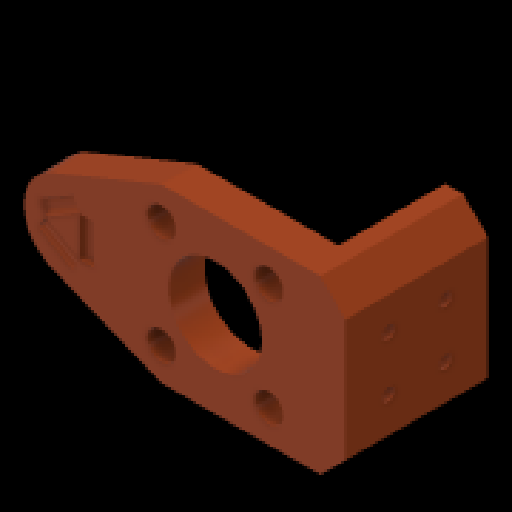
# Autodesk Inventor part: Rear Z Axis Carriage
Saved by Autodesk Inventor 2023.2 (Build 272271000, 271)
## iProperties
Created: 2023-02-17
Part Number: Rear Z Axis Carriage
Material: ABS Plastic
Document SubType Name: Modeling
Designer: remop
Density: 1.06 g/cm^3
Appearance: Smooth - Light Orange
Author: remop
Autodesk Inventor part; units mm, degrees
ref_plane "YZ Plane" through (0, 0, 0) normal (1, 0, 0) x (0, 1, 0)
ref_plane "XZ Plane" through (0, 0, 0) normal (0, 1, 0) x (-1, 0, 0)
ref_plane "XY Plane" through (0, 0, 0) normal (0, 0, 1) x (1, 0, 0)
sketch "Sketch1" plane through (0, 0, 0) normal (0, 0, 1) x (1, 0, 0)
  arc A0 (18.1843, -16.5324) -> (18.7618, -13.101) centre (16.0629, -14.4111) ccw projected
  arc A1 (18.7618, 13.101) -> (18.7618, -13.101) centre (45.75, 0) ccw projected
  arc A2 (18.7618, 13.101) -> (18.1843, 16.5324) centre (16.0629, 14.4111) ccw projected
  line L0 (11.5324, 23.1843) -> (18.1843, 16.5324) projected
  arc A3 (11.5324, 23.1843) -> (8.101, 23.7618) centre (9.4111, 21.0629) ccw projected
  arc A4 (-18.101, 23.7618) -> (8.101, 23.7618) centre (-5, 50.75) ccw projected
  arc A5 (-18.101, 23.7618) -> (-21.5324, 23.1843) centre (-19.4111, 21.0629) ccw projected
  line L1 (-28.1843, 16.5324) -> (-21.5324, 23.1843) projected
  arc A6 (-28.1843, 16.5324) -> (-28.7618, 13.101) centre (-26.0629, 14.4111) ccw projected
  arc A7 (-28.7618, -13.101) -> (-28.7618, 13.101) centre (-55.75, 0) ccw projected
  arc A8 (-28.7618, -13.101) -> (-28.1843, -16.5324) centre (-26.0629, -14.4111) ccw projected
  line L2 (-21.5324, -23.1843) -> (-28.1843, -16.5324) projected
  arc A9 (-21.5324, -23.1843) -> (-18.101, -23.7618) centre (-19.4111, -21.0629) ccw projected
  arc A10 (8.101, -23.7618) -> (-18.101, -23.7618) centre (-5, -50.75) ccw projected
  arc A11 (8.101, -23.7618) -> (11.5324, -23.1843) centre (9.4111, -21.0629) ccw projected
  line L3 (18.1843, -16.5324) -> (11.5324, -23.1843) projected
  circle A12 centre (10, -15) radius 4 projected
  circle A13 centre (-20, -15) radius 4 projected
  circle A14 centre (-20, 15) radius 4 projected
  circle A15 centre (10, 15) radius 4 projected
  circle A16 centre (-5, 0) radius 13 projected
  line L4 (39.4645, -4.5) -> (34.9645, -4.5) projected
  line L5 (34.9645, -4.5) -> (34.9645, 4.5) projected
  line L6 (34.9645, 4.5) -> (39.4645, 4.5) projected
  line L7 (39.4645, 4.5) -> (39.4645, 10) projected
  line L8 (39.4645, 10) -> (31.4645, 10) projected
  line L9 (31.4645, 10) -> (31.4645, -10) projected
  line L10 (31.4645, -10) -> (39.4645, -10) projected
  line L11 (39.4645, -10) -> (39.4645, -4.5) projected
  line L12 (31.4645, -10) -> (31.4645, -17.0711)
  line L13 (31.4645, -17.0711) -> (24.4726, -24.0629)
  line L14 (31.4645, 10) -> (31.4645, 17.0711)
  line L15 (-19.4111, -24.0629) -> (24.4726, -24.0629)
  line L16 (-19.4111, 24.0629) -> (24.4726, 24.0629)
  line L17 (31.4645, 17.0711) -> (24.4726, 24.0629)
  circle A17 centre (-46, 0) radius 12.5
  line L18 (-20.5407, -23.8421) -> (-50.7071, -11.5799)
  line L19 (-50.7071, 11.5799) -> (-20.5407, 23.8421)
  point P0 (0, 0)
  dimension "d0" = 45
  dimension "d1" = 5
  dimension "d4" = 46
  dimension "d5" = 25
  constraints: 16 end point, 8 tangent, 6 point on circle, 3 equal length, 2 vertical, 1 centre point, 1 horizontal alignment, 1 point on line
  measures "d0" angle of L12 L13
  measures "d1" distance from line of L9.end L13
  measures "d4" distance of A17.centre point (0, 0)
  measures "d5" diameter of A17
extrude "Extrusion1" add sketch "Sketch1" along normal blind 10 contours L3 A11 A10 A9 L2 A8 A7 A6 L1 A5 A4 A3 L0 A2 A1 A0 | A0 A1 A2 L0 A3 L16 L17 L14 L9 L12 L13 L15 A11 L3 | L15 A9 A10 A11 | L18 A17 L19 A5 L1 A6 A7 A8 L2 A9 | A3 A4 A5 L16 | A17
sketch "Sketch2" plane through (0, 0, 0) normal (0, 0, -1) x (-1, 0, 0)
  line L0 (-24.4726, -24.0629) -> (-31.4645, -17.0711) projected
  line L1 (19.4111, -24.0629) -> (-24.4726, -24.0629) projected
  arc A0 (19.4111, -24.0629) -> (20.5407, -23.8421) centre (19.4111, -21.0629) ccw projected
  line L2 (50.7071, -11.5799) -> (20.5407, -23.8421) projected
  arc A1 (50.7071, -11.5799) -> (50.7071, 11.5799) centre (46, 0) ccw projected
  line L3 (20.5407, 23.8421) -> (50.7071, 11.5799) projected
  arc A2 (20.5407, 23.8421) -> (19.4111, 24.0629) centre (19.4111, 21.0629) ccw projected
  line L4 (-24.4726, 24.0629) -> (19.4111, 24.0629) projected
  line L5 (-31.4645, 17.0711) -> (-24.4726, 24.0629) projected
  line L6 (-31.4645, -17.0711) -> (-31.4645, 17.0711) projected
  circle A3 centre (-10, -15) radius 4 projected
  circle A4 centre (20, -15) radius 4 projected
  circle A5 centre (20, 15) radius 4 projected
  circle A6 centre (-10, 15) radius 4 projected
  circle A7 centre (5, 0) radius 13 projected
  line L7 (-31.4645, 17.0711) -> (-23.4645, 17.0711)
  line L8 (-23.4645, 17.0711) -> (-23.4645, -17.0711)
  line L9 (-24.4726, -24.0629) -> (-31.4645, -17.0711) projected
  line L10 (-23.4645, -17.0711) -> (-31.4645, -17.0711)
  line L11 (-23.4645, 17.0711) -> (-19.4726, 21.0629)
  line L12 (-19.4726, 21.0629) -> (-19.4726, 24.0629)
  line L13 (-23.4645, -17.0711) -> (-19.4726, -21.0629)
  line L14 (-19.4726, -21.0629) -> (-19.4726, -24.0629)
  line L15 (19.4111, -24.0629) -> (-24.4726, -24.0629) projected
  point P0 (0, 0)
  dimension "d6" = 8
  dimension "d9" = 3
  constraints: 14 end point, 3 perpendicular, 3 point on line, 2 horizontal, 1 parallel, 1 vertical
  measures "d6" distance of L5.start L7.end
  measures "d9" distance of L11.end L12.end
extrude "Extrusion2" add sketch "Sketch2" along normal blind 29.9 contours L0 L10 L13 L14 L1 | L6 L7 L8 L10 | L5 L4 L12 L11 L7
sketch "Sketch3" plane through (23.4645, -17.0711, 0) normal (-1, 0, 0) x (0, 0, 1)
  line L0 (0, 34.1421) -> (0, 0) projected
  line L1 (0, 34.1421) -> (-29.9, 34.1421) projected
  line L2 (-29.9, 0) -> (-29.9, 34.1421) projected
  line L3 (0, 0) -> (-29.9, 0) projected
  point P0 (0, 17.0711)
  point P1 (-1.95, 25.0158)
  point P2 (-17.95, 25.0158)
  point P3 (-17.95, 10.0158)
  point P4 (-1.95, 10.0158)
  dimension "d10" = 15
  dimension "d11" = 16
  dimension "d12" = 11.95
  constraints: 2 horizontal alignment, 2 vertical alignment
  measures "d10" distance of point (-1.95, 10.016) point (-1.95, 25.016)
  measures "d11" distance of point (-17.95, 25.016) point (-1.95, 25.016)
  measures "d12" distance from line of L2 point (-17.95, 25.016)
hole "Hole1" at (23.4645, 7.9447, -1.95) at (23.4645, 7.9447, -17.95) at (23.4645, -7.0553, -17.95) at (23.4645, -7.0553, -1.95) direction (1, 0, 0) diameter 3.6 end through all counterbore diameter 6.5 counterbore depth 3.4 clearance for "Socket Head Cap Screw DIN EN ISO 4762" size "M3" standard "DIN"
sketch "Sketch4" plane through (0, 0, 0) normal (0, 0, -1) x (-1, 0, 0)
  circle A0 centre (5, 0) radius 13 projected
  circle A1 centre (-10, 15) radius 4 projected
  circle A2 centre (20, 15) radius 4 projected
  circle A3 centre (20, -15) radius 4 projected
  circle A4 centre (-10, -15) radius 4 projected
  line L0 (-19.4726, 24.0629) -> (-19.4726, 21.0629) projected
  line L1 (-19.4726, 21.0629) -> (-23.4645, 17.0711) projected
  line L2 (-23.4645, 17.0711) -> (-23.4645, 10.5447) projected
  line L3 (-23.4645, 10.5447) -> (-23.4645, 5.3447) projected
  line L4 (-23.4645, 5.3447) -> (-23.4645, -4.4553) projected
  line L5 (-23.4645, -4.4553) -> (-23.4645, -9.6553) projected
  line L6 (-23.4645, -9.6553) -> (-23.4645, -17.0711) projected
  line L7 (-23.4645, -17.0711) -> (-19.4726, -21.0629) projected
  line L8 (-19.4726, -21.0629) -> (-19.4726, -24.0629) projected
  line L9 (19.4111, -24.0629) -> (-19.4726, -24.0629) projected
  arc A5 (19.4111, -24.0629) -> (20.5407, -23.8421) centre (19.4111, -21.0629) ccw projected
  line L10 (50.7071, -11.5799) -> (20.5407, -23.8421) projected
  arc A6 (50.7071, -11.5799) -> (50.7071, 11.5799) centre (46, 0) ccw projected
  line L11 (20.5407, 23.8421) -> (50.7071, 11.5799) projected
  arc A7 (20.5407, 23.8421) -> (19.4111, 24.0629) centre (19.4111, 21.0629) ccw projected
  line L12 (-19.4726, 24.0629) -> (19.4111, 24.0629) projected
  line L13 (-19.4726, 21.0629) -> (-15.4807, 17.0711)
  line L14 (-15.4807, 17.0711) -> (-15.4807, -17.0711)
  line L15 (-15.4807, -17.0711) -> (-19.4726, -21.0629)
  line L16 (-23.4645, 17.0711) -> (-19.4726, 21.0629) projected
  point P0 (0, 0)
  constraints: 6 end point, 3 perpendicular, 1 vertical
extrude "Extrusion3" cut sketch "Sketch4" against normal blind 2 contours L13 L14 L15 L7 L6 L5 L4 L3 L2 L1
sketch "Sketch6" plane through (0, 0, 10) normal (0, 0, 1) x (1, 0, 0)
  line L0 (24.4726, -24.0629) -> (31.4645, -17.0711) projected
  line L1 (31.4645, -17.0711) -> (31.4645, 17.0711) projected
  line L2 (31.4645, 17.0711) -> (24.4726, 24.0629) projected
  line L3 (24.4726, 24.0629) -> (-19.4111, 24.0629) projected
  arc A0 (-19.4111, 24.0629) -> (-20.5407, 23.8421) centre (-19.4111, 21.0629) ccw projected
  line L4 (-20.5407, 23.8421) -> (-50.7071, 11.5799) projected
  arc A1 (-50.7071, 11.5799) -> (-50.7071, -11.5799) centre (-46, 0) ccw projected
  line L5 (-50.7071, -11.5799) -> (-20.5407, -23.8421) projected
  arc A2 (-20.5407, -23.8421) -> (-19.4111, -24.0629) centre (-19.4111, -21.0629) ccw projected
  line L6 (-19.4111, -24.0629) -> (24.4726, -24.0629) projected
  circle A3 centre (10, -15) radius 4 projected
  circle A4 centre (-20, -15) radius 4 projected
  circle A5 centre (-20, 15) radius 4 projected
  circle A6 centre (10, 15) radius 4 projected
  circle A7 centre (-5, 0) radius 13 projected
  line L7 (-42.8246, 5.5) -> (-42.8246, -5.5)
  line L8 (-42.8246, -5.5) -> (-52.3509, 0)
  line L9 (-52.3509, 0) -> (-42.8246, 5.5)
  line L10 (-42.8246, 0) -> (-46, 0) construction
  line L11 (-46, 0) -> (-47.5877, 2.75) construction
  line L12 (-46, 0) -> (-47.5877, -2.75) construction
  line L13 (-52.3509, 0) -> (-54.3509, 3.4641)
  line L14 (-54.3509, 3.4641) -> (-44.8246, 8.9641)
  line L15 (-44.8246, 8.9641) -> (-42.8246, 5.5)
  line L16 (-42.8246, 5.5) -> (-38.8246, 5.5)
  line L17 (-38.8246, 5.5) -> (-38.8246, -5.5)
  line L18 (-38.8246, -5.5) -> (-42.8246, -5.5)
  line L19 (-42.8246, -5.5) -> (-44.8246, -8.9641)
  line L20 (-44.8246, -8.9641) -> (-54.3509, -3.4641)
  line L21 (-54.3509, -3.4641) -> (-52.3509, 0)
  line L22 (-43.1308, 5.3232) -> (-43.0014, 5.8062)
  line L23 (-42.471, 5.5) -> (-42.8246, 5.1464)
  line L24 (-42.471, -5.5) -> (-42.8246, -5.1464)
  line L25 (-43.1308, -5.3232) -> (-43.0014, -5.8062)
  line L26 (-52.0447, -0.1768) -> (-52.5276, -0.3062)
  line L27 (-52.0447, 0.1768) -> (-52.5276, 0.3062)
  point P0 (0, 0)
  dimension "d27" = 11
  dimension "d28" = 4
  dimension "d33" = 45
  dimension "d34" = 45
  dimension "d35" = 45
  dimension "d36" = 45
  dimension "d37" = 45
  dimension "d38" = 135
  dimension "d39" = 0.5
  constraints: 42 end point, 13 point on line, 10 equal length, 5 perpendicular, 3 horizontal, 3 midpoint, 2 parallel, 1 coincident, 1 horizontal alignment, 1 vertical
  measures "d27" distance of L7.start L7.end
  measures "d28" distance of L17.end L18.end
  measures "d33" angle of L23 L7
  measures "d34" angle of L9 L22
  measures "d35" angle of L9 L27
  measures "d36" angle of L8 L26
  measures "d37" angle of L8 L25
  measures "d38" angle of L7 L24
  measures "d39" distance of L24.start L24.end
extrude "Extrusion5" cut sketch "Sketch6" against normal blind 1.5 contours L23 L16 L17 L18 L24 L7 | L9 L27 L13 L14 L15 L22 | L25 L19 L20 L21 L26 L8
fillet "Fillet2" radius 2 6 edges at (-47.5877, 2.75, 8.5) (-49.5877, 6.2141, 8.5) (-38.8246, 0, 8.5) (-42.8246, 0, 8.5) (-47.5877, -2.75, 8.5) (-49.5877, -6.2141, 8.5)
sketch "Sketch7" plane through (0, 0, 0) normal (0, 0, -1) x (-1, 0, 0)
  line L0 (-19.4726, 21.0629) -> (-15.4807, 17.0711) projected
  line L1 (-15.4807, 17.0711) -> (-15.4807, -17.0711) projected
  line L2 (-15.4807, -17.0711) -> (-19.4726, -21.0629) projected
  line L3 (-19.4726, -21.0629) -> (-19.4726, -24.0629) projected
  line L4 (19.4111, -24.0629) -> (-19.4726, -24.0629) projected
  arc A0 (19.4111, -24.0629) -> (20.5407, -23.8421) centre (19.4111, -21.0629) ccw projected
  line L5 (50.7071, -11.5799) -> (20.5407, -23.8421) projected
  arc A1 (50.7071, -11.5799) -> (50.7071, 11.5799) centre (46, 0) ccw projected
  line L6 (20.5407, 23.8421) -> (50.7071, 11.5799) projected
  arc A2 (20.5407, 23.8421) -> (19.4111, 24.0629) centre (19.4111, 21.0629) ccw projected
  line L7 (-19.4726, 24.0629) -> (19.4111, 24.0629) projected
  line L8 (-19.4726, 24.0629) -> (-19.4726, 21.0629) projected
  circle A3 centre (-10, -15) radius 4 projected
  circle A4 centre (20, -15) radius 4 projected
  circle A5 centre (20, 15) radius 4 projected
  circle A6 centre (-10, 15) radius 4 projected
  circle A7 centre (5, 0) radius 13 projected
  line L9 (-13.8891, 21.7175) -> (-3.2825, 11.1109)
  line L10 (-3.2825, 11.1109) -> (-1.1612, 13.2322)
  line L11 (-1.1612, 13.2322) -> (-11.7678, 23.8388)
  line L12 (-11.7678, 23.8388) -> (-13.8891, 21.7175)
  line L13 (-6.1109, 8.2825) -> (-16.7175, 18.8891)
  line L14 (-16.7175, 18.8891) -> (-18.8388, 16.7678)
  line L15 (-18.8388, 16.7678) -> (-8.2322, 6.1612)
  line L16 (-8.2322, 6.1612) -> (-6.1109, 8.2825)
  line L17 (-10, 15) -> (-8.5858, 16.4142) construction
  line L18 (-10, 15) -> (-11.4142, 13.5858) construction
  line L19 (11.1612, -13.2322) -> (21.7678, -23.8388)
  line L20 (21.7678, -23.8388) -> (23.8891, -21.7175)
  line L21 (23.8891, -21.7175) -> (13.2825, -11.1109)
  line L22 (13.2825, -11.1109) -> (11.1612, -13.2322)
  line L23 (18.2322, -6.1612) -> (16.1109, -8.2825)
  line L24 (16.1109, -8.2825) -> (26.7175, -18.8891)
  line L25 (26.7175, -18.8891) -> (28.8388, -16.7678)
  line L26 (28.8388, -16.7678) -> (18.2322, -6.1612)
  point P0 (0, 0)
  point P1 (18.5858, -16.4142)
  point P2 (21.4142, -13.5858)
  point P3 (21.4155, -23.4865)
  point P4 (22.6026, -23.004)
  point P5 (21.0353, -18.8637)
  point P6 (16.1363, -13.9647)
  point P7 (18.9647, -11.1363)
  point P8 (23.8637, -16.0353)
  point P9 (-11.0353, 18.8637)
  point P10 (-6.1363, 13.9647)
  point P11 (-8.9647, 11.1363)
  point P12 (-13.8637, 16.0353)
  point P13 (-17.0081, 18.5985)
  point P14 (-15.4807, 13.4097)
  dimension "d41" = 45
  dimension "d42" = 3
  dimension "d43" = 15
  dimension "d44" = 4
  dimension "d47" = 360
  constraints: 36 end point, 5 parallel, 4 perpendicular, 3 equal length, 3 midpoint, 2 point on line, 37 other
  measures "d41" angle of L7 L11
  measures "d42" distance of L9.end L10.end
  measures "d43" distance of L10.end L11.end
  measures "d44" distance between parallel lines of L13 L9
extrude "Extrusion6" cut sketch "Sketch7" against normal blind 1.5 contours L14 L13 A6 L16 L15 L1 L0 | L9 L12 L11 L10 A6 | L5 L19 L22 L21 A4 L20 | A4 L24 L23 L26 L25
fillet "Fillet3" radius 1.5 12 edges at (12.4622, 20.2906, 1.5) (6.4645, 18.5355, 1.5) (4.7094, 12.5378, 1.5) (11.8565, 9.7854, 1.5) (7.5378, 9.7094, 1.5) (15.2906, 17.4622, 1.5) (-16.2883, -18.3594, 1.5) (-14.7094, -12.5378, 1.5) (-17.5378, -9.7094, 1.5) (-23.5355, -11.4645, 1.5) (-25.2906, -17.4622, 1.5) (-22.4622, -20.2906, 1.5)
sketch "Sketch8" plane through (0, 0, 10) normal (0, 0, 1) x (1, 0, 0)
  line L0 (-42.8246, 5.1464) -> (-42.471, 5.5) projected
  line L1 (-42.471, 5.5) -> (-38.8246, 5.5) projected
  line L2 (-38.8246, 5.5) -> (-38.8246, -5.5) projected
  line L3 (-38.8246, -5.5) -> (-42.471, -5.5) projected
  line L4 (-42.471, -5.5) -> (-42.8246, -5.1464) projected
  line L5 (-42.8246, -5.1464) -> (-42.8246, 5.1464) projected
  line L6 (-43.1308, -5.3232) -> (-43.0014, -5.8062) projected
  line L7 (-43.0014, -5.8062) -> (-44.8246, -8.9641) projected
  line L8 (-44.8246, -8.9641) -> (-54.3509, -3.4641) projected
  line L9 (-54.3509, -3.4641) -> (-52.5276, -0.3062) projected
  line L10 (-52.5276, -0.3062) -> (-52.0447, -0.1768) projected
  line L11 (-52.0447, -0.1768) -> (-43.1308, -5.3232) projected
  line L12 (-52.0447, 0.1768) -> (-52.5276, 0.3062) projected
  line L13 (-52.5276, 0.3062) -> (-54.3509, 3.4641) projected
  line L14 (-54.3509, 3.4641) -> (-44.8246, 8.9641) projected
  line L15 (-44.8246, 8.9641) -> (-43.0014, 5.8062) projected
  line L16 (-43.0014, 5.8062) -> (-43.1308, 5.3232) projected
  line L17 (-43.1308, 5.3232) -> (-52.0447, 0.1768) projected
  line L18 (24.4726, -24.0629) -> (31.4645, -17.0711) projected
  line L19 (31.4645, -17.0711) -> (31.4645, 17.0711) projected
  line L20 (31.4645, 17.0711) -> (24.4726, 24.0629) projected
  line L21 (24.4726, 24.0629) -> (-19.4111, 24.0629) projected
  arc A0 (-19.4111, 24.0629) -> (-20.5407, 23.8421) centre (-19.4111, 21.0629) ccw projected
  line L22 (-20.5407, 23.8421) -> (-50.7071, 11.5799) projected
  arc A1 (-50.7071, 11.5799) -> (-50.7071, -11.5799) centre (-46, 0) ccw projected
  line L23 (-50.7071, -11.5799) -> (-20.5407, -23.8421) projected
  arc A2 (-20.5407, -23.8421) -> (-19.4111, -24.0629) centre (-19.4111, -21.0629) ccw projected
  line L24 (-19.4111, -24.0629) -> (24.4726, -24.0629) projected
  circle A3 centre (10, -15) radius 4 projected
  circle A4 centre (-20, -15) radius 4 projected
  circle A5 centre (-20, 15) radius 4 projected
  circle A6 centre (10, 15) radius 4 projected
  circle A7 centre (-5, 0) radius 13 projected
  point P0 (0, 0)
extrude "Extrusion7" add sketch "Sketch8" against normal blind 1.5 contours A3 | A4 | A5 | A6
sketch "Sketch9" plane through (0, 0, 0) normal (0, 0, -1) x (-1, 0, 0)
  circle A0 centre (-10, -15) radius 4 projected
  circle A1 centre (20, 15) radius 4 projected
  point P0 (0, 0)
extrude "Extrusion8" add sketch "Sketch9" against normal up to surface (8.5 mm away)
sketch "Sketch10" plane through (0, 0, 0) normal (0, 0, -1) x (-1, 0, 0)
  circle A0 centre (5, 0) radius 13 projected
  line L0 (18.9647, -11.1363) -> (16.1109, -8.2825) projected
  line L1 (16.1109, -8.2825) -> (18.2322, -6.1612) projected
  line L2 (18.2322, -6.1612) -> (28.8388, -16.7678) projected
  line L3 (28.8388, -16.7678) -> (26.7175, -18.8891) projected
  line L4 (26.7175, -18.8891) -> (23.8637, -16.0353) projected
  arc A1 (21.0353, -18.8637) -> (23.8637, -16.0353) centre (20, -15) ccw projected
  line L5 (21.0353, -18.8637) -> (23.8891, -21.7175) projected
  line L6 (23.8891, -21.7175) -> (22.6026, -23.004) projected
  line L7 (50.7071, -11.5799) -> (22.6026, -23.004) projected
  arc A2 (50.7071, -11.5799) -> (50.7071, 11.5799) centre (46, 0) ccw projected
  line L8 (20.5407, 23.8421) -> (50.7071, 11.5799) projected
  arc A3 (20.5407, 23.8421) -> (19.4111, 24.0629) centre (19.4111, 21.0629) ccw projected
  line L9 (-19.4726, 24.0629) -> (19.4111, 24.0629) projected
  line L10 (-19.4726, 24.0629) -> (-19.4726, 21.0629) projected
  line L11 (-19.4726, 21.0629) -> (-17.0081, 18.5985) projected
  line L12 (-17.0081, 18.5985) -> (-16.7175, 18.8891) projected
  line L13 (-16.7175, 18.8891) -> (-13.8637, 16.0353) projected
  arc A4 (-11.0353, 18.8637) -> (-13.8637, 16.0353) centre (-10, 15) ccw projected
  line L14 (-11.0353, 18.8637) -> (-13.8891, 21.7175) projected
  line L15 (-13.8891, 21.7175) -> (-11.7678, 23.8388) projected
  line L16 (-11.7678, 23.8388) -> (-1.1612, 13.2322) projected
  line L17 (-1.1612, 13.2322) -> (-3.2825, 11.1109) projected
  line L18 (-3.2825, 11.1109) -> (-6.1363, 13.9647) projected
  arc A5 (-8.9647, 11.1363) -> (-6.1363, 13.9647) centre (-10, 15) ccw projected
  line L19 (-8.9647, 11.1363) -> (-6.1109, 8.2825) projected
  line L20 (-6.1109, 8.2825) -> (-8.2322, 6.1612) projected
  line L21 (-8.2322, 6.1612) -> (-15.4807, 13.4097) projected
  line L22 (-15.4807, 13.4097) -> (-15.4807, -17.0711) projected
  line L23 (-15.4807, -17.0711) -> (-19.4726, -21.0629) projected
  line L24 (-19.4726, -21.0629) -> (-19.4726, -24.0629) projected
  line L25 (19.4111, -24.0629) -> (-19.4726, -24.0629) projected
  arc A6 (19.4111, -24.0629) -> (20.5407, -23.8421) centre (19.4111, -21.0629) ccw projected
  line L26 (21.4155, -23.4865) -> (20.5407, -23.8421) projected
  line L27 (21.4155, -23.4865) -> (11.1612, -13.2322) projected
  line L28 (11.1612, -13.2322) -> (13.2825, -11.1109) projected
  line L29 (13.2825, -11.1109) -> (16.1363, -13.9647) projected
  arc A7 (18.9647, -11.1363) -> (16.1363, -13.9647) centre (20, -15) ccw projected
  circle A8 centre (46, 0) radius 4.5
  circle A9 centre (5, 0) radius 23
  line L30 (47.6945, 4.1688) -> (23.1288, 14.1544)
  line L31 (47.6945, -4.1688) -> (23.1288, -14.1544)
  line L32 (50.7071, -11.5799) -> (22.6026, -23.004) projected
  line L33 (20.5407, 23.8421) -> (50.7071, 11.5799) projected
  line L34 (26.3306, -8.6027) -> (29.3525, -11.6246)
  point P0 (0, 0)
  dimension "d56" = 8
  dimension "d57" = 10
  dimension "d58" = 4
  constraints: 6 end point, 5 point on circle, 3 parallel, 2 centre point, 2 coincident, 2 tangent, 1 point on line
  measures "d56" radial gap between concentric circles of A2 A8
  measures "d57" radial gap between concentric circles of A9 A0
  measures "d58" distance between parallel lines of L2 L34
extrude "Extrusion9" cut sketch "Sketch10" against normal blind 7 contours A9 L30 A8 L31 L34 | A8
fillet "Fillet4" radius 2 3 edges at (-23.1288, 14.1544, 3.5) (-26.3306, -8.6027, 3.5) (-29.3525, -11.6246, 3.5)
chamfer "Chamfer1" distance 2 angle 45 8 edges at (-27.9795, 0.9705, 0) (-26.4518, 11.456, 0) (-38.1667, 8.0417, 0) (-50.5, 0, 0) (-39.1381, -7.6468, 0) (-29.4318, -11.2324, 0) (-27.8264, -10.0985, 0) (-26.7044, -8.548, 0)
equation "\"d34\" = d33"
equation "\"d36\" = d35"
equation "\"d37\" = d36"
equation "\"d58\" = 0.5 * d56"
body "Solid1"
